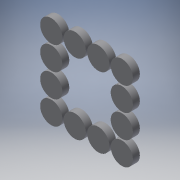
# Autodesk Inventor part: WeightCap
Saved by Autodesk Inventor 2019.3 (Build 233278000, 278)
## iProperties
Created: 2019-07-14
Part Number: WeightCap
Material: Generic
Document SubType Name: Modeling
Designer: mark
Density: 1 g/cm^3
Appearance: Default
Author: mark
Autodesk Inventor part; units mm, degrees
ref_plane "YZ Plane" through (0, 0, 0) normal (1, 0, 0) x (0, 1, 0)
ref_plane "XZ Plane" through (0, 0, 0) normal (0, 1, 0) x (-1, 0, 0)
ref_plane "XY Plane" through (0, 0, 0) normal (0, 0, 1) x (1, 0, 0)
sketch "Sketch1" plane through (0, 0, 0) normal (0, 0, 1) x (1, 0, 0)
  circle A0 centre (16.335, -16.335) radius 2.25 projected
  circle A1 centre (-16.335, 16.335) radius 2.25 projected
  circle A2 centre (16.335, 16.335) radius 2.25 projected
  circle A3 centre (-16.335, -16.335) radius 2.25 projected
  line L0 (-13.335, 13.335) -> (13.335, 13.335) projected
  line L1 (13.335, 13.335) -> (13.335, -13.335) projected
  line L2 (13.335, -13.335) -> (-13.335, -13.335) projected
  line L3 (-13.335, -13.335) -> (-13.335, 13.335) projected
  circle A4 centre (25.5, -25.5) radius 8.0375 projected
  circle A5 centre (8.5, -25.5) radius 8.0375 projected
  circle A6 centre (-25.5, -25.5) radius 8.0375 projected
  circle A7 centre (-8.5, -25.5) radius 8.0375 projected
  circle A8 centre (25.5, -8.5) radius 8.0375 projected
  circle A9 centre (25.5, 8.5) radius 8.0375 projected
  circle A10 centre (-25.5, -8.5) radius 8.0375 projected
  circle A11 centre (-25.5, 8.5) radius 8.0375 projected
  circle A12 centre (25.5, 25.5) radius 8.0375 projected
  circle A13 centre (8.5, 25.5) radius 8.0375 projected
  circle A14 centre (-25.5, 25.5) radius 8.0375 projected
  circle A15 centre (-8.5, 25.5) radius 8.0375 projected
  arc A16 (29.5, -34.5) -> (34.5, -29.5) centre (29.5, -29.5) ccw projected
  line L4 (34.5, -29.5) -> (34.5, 29.5) projected
  arc A17 (34.5, 29.5) -> (29.5, 34.5) centre (29.5, 29.5) ccw projected
  line L5 (29.5, 34.5) -> (-29.5, 34.5) projected
  arc A18 (-29.5, 34.5) -> (-34.5, 29.5) centre (-29.5, 29.5) ccw projected
  line L6 (-34.5, 29.5) -> (-34.5, -29.5) projected
  arc A19 (-34.5, -29.5) -> (-29.5, -34.5) centre (-29.5, -29.5) ccw projected
  line L7 (-29.5, -34.5) -> (29.5, -34.5) projected
  point P0 (0, 0)
extrude "Extrusion1" add sketch "Sketch1" against normal blind 5 contours A4 | A5 | A6 | A7 | A8 | A9 | A10 | A11 | A12 | A13 | A14 | A15
ref_plane "Work Plane1" through (0, 0, 0) normal (0, 0, 1) x (1, 0, 0)
sketch "Sketch2" plane through (0, 0, 0) normal (0, 0, 1) x (1, 0, 0)
  circle A0 centre (16.335, -16.335) radius 2.25 projected
  circle A1 centre (-16.335, 16.335) radius 2.25 projected
  circle A2 centre (16.335, 16.335) radius 2.25 projected
  circle A3 centre (-16.335, -16.335) radius 2.25 projected
  line L0 (-13.335, 13.335) -> (13.335, 13.335) projected
  line L1 (13.335, 13.335) -> (13.335, -13.335) projected
  line L2 (13.335, -13.335) -> (-13.335, -13.335) projected
  line L3 (-13.335, -13.335) -> (-13.335, 13.335) projected
  circle A4 centre (25.5, -25.5) radius 8.0375 projected
  circle A5 centre (8.5, -25.5) radius 8.0375 projected
  circle A6 centre (-25.5, -25.5) radius 8.0375 projected
  circle A7 centre (-8.5, -25.5) radius 8.0375 projected
  circle A8 centre (25.5, -8.5) radius 8.0375 projected
  circle A9 centre (25.5, 8.5) radius 8.0375 projected
  circle A10 centre (-25.5, -8.5) radius 8.0375 projected
  circle A11 centre (-25.5, 8.5) radius 8.0375 projected
  circle A12 centre (25.5, 25.5) radius 8.0375 projected
  circle A13 centre (8.5, 25.5) radius 8.0375 projected
  circle A14 centre (-25.5, 25.5) radius 8.0375 projected
  circle A15 centre (-8.5, 25.5) radius 8.0375 projected
  arc A16 (29.5, -34.5) -> (34.5, -29.5) centre (29.5, -29.5) ccw projected
  line L4 (34.5, -29.5) -> (34.5, 29.5) projected
  arc A17 (34.5, 29.5) -> (29.5, 34.5) centre (29.5, 29.5) ccw projected
  line L5 (29.5, 34.5) -> (-29.5, 34.5) projected
  arc A18 (-29.5, 34.5) -> (-34.5, 29.5) centre (-29.5, 29.5) ccw projected
  line L6 (-34.5, 29.5) -> (-34.5, -29.5) projected
  arc A19 (-34.5, -29.5) -> (-29.5, -34.5) centre (-29.5, -29.5) ccw projected
  line L7 (-29.5, -34.5) -> (29.5, -34.5) projected
  circle A20 centre (-16.335, 16.335) radius 3.25
  circle A21 centre (16.335, 16.335) radius 3.25
  circle A22 centre (-16.335, -16.335) radius 3.25
  circle A23 centre (16.335, -16.335) radius 3.25
  point P0 (0, 0)
  dimension "d4" = 1
  dimension "d5" = 1
  dimension "d6" = 1
  dimension "d7" = 1
  constraints: 4 centre point
  measures "d4" radial gap between concentric circles of A1 A20
  measures "d5" radial gap between concentric circles of A2 A21
  measures "d6" radial gap between concentric circles of A3 A22
  measures "d7" radial gap between concentric circles of A0 A23
extrude "Extrusion2" add sketch "Sketch2" along normal blind 15 contours A4 | A5 | A6 | A7 | A8 | A9 | A10 | A11 | A12 | A13 | A14 | A15 | L7 A19 L6 A18 L5 A17 L4 A16
sketch "Sketch3" plane through (25.5, 25.5, -5) normal (0, 0, -1) x (-1, 0, 0)
  line L0 (-4.0375, 2.0375) -> (-2.0375, 2.0375)
  line L1 (-2.0375, 2.0375) -> (-2.0375, -2.0375)
  line L2 (-2.0375, -2.0375) -> (-4.0375, -2.0375)
  line L3 (-4.0375, -2.0375) -> (-4.0375, 2.0375)
  circle A0 centre (0, 0) radius 8.0375 projected
  line L4 (12.165, -12.165) -> (38.835, -12.165) projected
  line L5 (12.165, -38.835) -> (12.165, -12.165) projected
  line L6 (12.9625, 2.0375) -> (14.9625, 2.0375)
  line L7 (14.9625, 2.0375) -> (14.9625, -2.0375)
  line L8 (14.9625, -2.0375) -> (12.9625, -2.0375)
  line L9 (12.9625, -2.0375) -> (12.9625, 2.0375)
  line L10 (29.9625, 2.0375) -> (31.9625, 2.0375)
  line L11 (31.9625, 2.0375) -> (31.9625, -2.0375)
  line L12 (31.9625, -2.0375) -> (29.9625, -2.0375)
  line L13 (29.9625, -2.0375) -> (29.9625, 2.0375)
  line L14 (46.9625, 2.0375) -> (48.9625, 2.0375)
  line L15 (48.9625, 2.0375) -> (48.9625, -2.0375)
  line L16 (48.9625, -2.0375) -> (46.9625, -2.0375)
  line L17 (46.9625, -2.0375) -> (46.9625, 2.0375)
  line L18 (-4.0375, -14.9625) -> (-2.0375, -14.9625)
  line L19 (-2.0375, -14.9625) -> (-2.0375, -19.0375)
  line L20 (-2.0375, -19.0375) -> (-4.0375, -19.0375)
  line L21 (-4.0375, -19.0375) -> (-4.0375, -14.9625)
  line L22 (12.9625, -14.9625) -> (14.9625, -14.9625)
  line L23 (14.9625, -14.9625) -> (14.9625, -19.0375)
  line L24 (14.9625, -19.0375) -> (12.9625, -19.0375)
  line L25 (12.9625, -19.0375) -> (12.9625, -14.9625)
  line L26 (29.9625, -14.9625) -> (31.9625, -14.9625)
  line L27 (31.9625, -14.9625) -> (31.9625, -19.0375)
  line L28 (31.9625, -19.0375) -> (29.9625, -19.0375)
  line L29 (29.9625, -19.0375) -> (29.9625, -14.9625)
  line L30 (46.9625, -14.9625) -> (48.9625, -14.9625)
  line L31 (48.9625, -14.9625) -> (48.9625, -19.0375)
  line L32 (48.9625, -19.0375) -> (46.9625, -19.0375)
  line L33 (46.9625, -19.0375) -> (46.9625, -14.9625)
  line L34 (-4.0375, -31.9625) -> (-2.0375, -31.9625)
  line L35 (-2.0375, -31.9625) -> (-2.0375, -36.0375)
  line L36 (-2.0375, -36.0375) -> (-4.0375, -36.0375)
  line L37 (-4.0375, -36.0375) -> (-4.0375, -31.9625)
  line L38 (12.9625, -31.9625) -> (14.9625, -31.9625)
  line L39 (14.9625, -31.9625) -> (14.9625, -36.0375)
  line L40 (14.9625, -36.0375) -> (12.9625, -36.0375)
  line L41 (12.9625, -36.0375) -> (12.9625, -31.9625)
  line L42 (29.9625, -31.9625) -> (31.9625, -31.9625)
  line L43 (31.9625, -31.9625) -> (31.9625, -36.0375)
  line L44 (31.9625, -36.0375) -> (29.9625, -36.0375)
  line L45 (29.9625, -36.0375) -> (29.9625, -31.9625)
  line L46 (46.9625, -31.9625) -> (48.9625, -31.9625)
  line L47 (48.9625, -31.9625) -> (48.9625, -36.0375)
  line L48 (48.9625, -36.0375) -> (46.9625, -36.0375)
  line L49 (46.9625, -36.0375) -> (46.9625, -31.9625)
  line L50 (-4.0375, -48.9625) -> (-2.0375, -48.9625)
  line L51 (-2.0375, -48.9625) -> (-2.0375, -53.0375)
  line L52 (-2.0375, -53.0375) -> (-4.0375, -53.0375)
  line L53 (-4.0375, -53.0375) -> (-4.0375, -48.9625)
  line L54 (12.9625, -48.9625) -> (14.9625, -48.9625)
  line L55 (14.9625, -48.9625) -> (14.9625, -53.0375)
  line L56 (14.9625, -53.0375) -> (12.9625, -53.0375)
  line L57 (12.9625, -53.0375) -> (12.9625, -48.9625)
  line L58 (29.9625, -48.9625) -> (31.9625, -48.9625)
  line L59 (31.9625, -48.9625) -> (31.9625, -53.0375)
  line L60 (31.9625, -53.0375) -> (29.9625, -53.0375)
  line L61 (29.9625, -53.0375) -> (29.9625, -48.9625)
  line L62 (46.9625, -48.9625) -> (48.9625, -48.9625)
  line L63 (48.9625, -48.9625) -> (48.9625, -53.0375)
  line L64 (48.9625, -53.0375) -> (46.9625, -53.0375)
  line L65 (46.9625, -53.0375) -> (46.9625, -48.9625)
  dimension "d9" = 2
  dimension "d10" = 6
  dimension "d11" = 6
  dimension "d12" = 4
  dimension "d15" = 17
  dimension "d18" = 17
  constraints: 128 end point, 3 horizontal, 2 vertical, 120 other
  measures "d9" distance between parallel lines of L3 L1
  measures "d10" distance edge to line of A0 L2
  measures "d11" distance edge to line of A0 L0
  measures "d12" distance edge to line of A0 L3
  measures "d15" distance of L0.start L6.start
  measures "d18" distance of L0.start L18.start
sketch "Sketch4" plane through (8.5, 25.5, -5) normal (0, 0, -1) x (-1, 0, 0)
  point P0 (8.5, -25.5)
ref_plane "Work Plane2" through (-34.5, -34.5, -179.8) normal (0, -1, 0) x (1, 0, 0)
sketch "Sketch5" plane through (-34.5, -34.5, -179.8) normal (0, -1, 0) x (1, 0, 0)
  line L0 (62.0375, 174.8) -> (64.0375, 174.8) projected
  line L1 (62.0375, 174.8) -> (57.0375, 169.8)
  line L2 (62.0375, 174.8) -> (69.1086, 174.8) construction
  point P0 (34.5, 179.8)
  dimension "d21" = 135
  dimension "d23" = 5
  constraints: 4 end point, 1 equal length, 1 horizontal
  measures "d21" angle of L1 L2
  measures "d23" horizontal distance of L0.start L1.end
sweep "Sweep1" add profiles "Sketch3" path "Sketch5" keep normal constant yes path curves L1 contours L0 L1 L2 L3 | L6 L7 L8 L9 | L10 L11 L12 L13 | L14 L15 L16 L17 | L18 L19 L20 L21 | L30 L31 L32 L33 | L34 L35 L36 L37 | L46 L47 L48 L49 | L50 L51 L52 L53 | L54 L55 L56 L57 | L58 L59 L60 L61 | L62 L63 L64 L65
sketch "Sketch6" plane through (-29.5, -34.5, 0) normal (0, -1, 0) x (1, 0, 0)
  circle A0 centre (29.5, 7.5) radius 6.75
  line L0 (59, 0) -> (0, 0) projected
  line L1 (64, 0) -> (64, 15) projected
  point P0 (29.5, 0)
  dimension "d26" = 7.5
  dimension "d27" = 13.5
  dimension "d28" = 34.5
  constraints: 1 centre point
  measures "d26" distance from line of L0 A0.centre
  measures "d27" diameter of A0
  measures "d28" distance from line of L1 A0.centre
extrude "Extrusion3" cut sketch "Sketch6" against normal blind 12
sketch "Sketch7" plane through (0, -22.5, 7.5) normal (0, -1, 0) x (1, 0, 0)
  circle A0 centre (0, 0) radius 6.75 projected
  circle A1 centre (0, 0) radius 4
  point P0 (0, -7.5)
  dimension "d31" = 8
  constraints: 1 centre point, 1 coincident
  measures "d31" diameter of A1
extrude "Extrusion4" cut sketch "Sketch7" against normal up to next contours A1
sketch "Sketch8" plane through (0, 0, 15) normal (0, 0, 1) x (1, 0, 0)
  circle A0 centre (16.335, 16.335) radius 3.25 projected
  circle A1 centre (16.335, -16.335) radius 3.25 projected
  circle A2 centre (-16.335, -16.335) radius 3.25 projected
  circle A3 centre (-16.335, 16.335) radius 3.25 projected
  circle A4 centre (16.335, 16.335) radius 4.35
  circle A5 centre (16.335, -16.335) radius 4.35
  circle A6 centre (-16.335, 16.335) radius 4.35
  circle A7 centre (-16.335, -16.335) radius 4.35
  point P0 (0, 0)
  dimension "d34" = 1.1
  dimension "d35" = 1.1
  dimension "d36" = 1.1
  dimension "d37" = 1.1
  constraints: 4 centre point
  measures "d34" radial gap between concentric circles of A0 A4
  measures "d35" radial gap between concentric circles of A1 A5
  measures "d36" radial gap between concentric circles of A3 A6
  measures "d37" radial gap between concentric circles of A2 A7
extrude "Extrusion5" cut sketch "Sketch8" against normal blind 5.2
body "Solid1"
